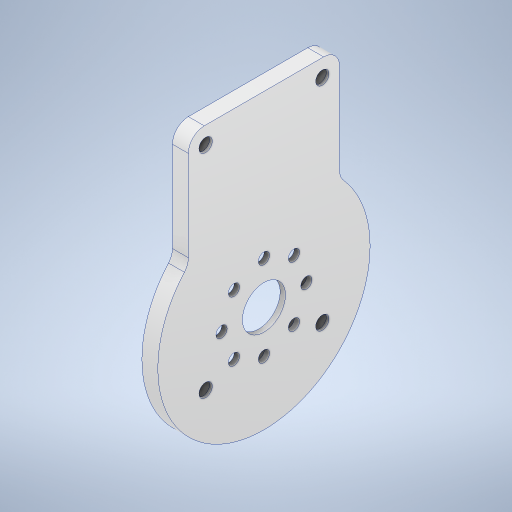
# Autodesk Inventor part: connectpart5
Saved by Autodesk Inventor 2024.3 (Build 283343010, 343A)
## iProperties
Created: 2025-06-29
Part Number: connectpart5
Material: アルミニウム 6061
Document SubType Name: Modeling
Designer: kshau
Density: 2.7 g/cm^3
Appearance: アルミニウム - フラット
Author: kshau
Autodesk Inventor part; units mm, degrees
ref_plane "YZ Plane" through (0, 0, 0) normal (1, 0, 0) x (0, 1, 0)
ref_plane "XZ Plane" through (0, 0, 0) normal (0, 1, 0) x (-1, 0, 0)
ref_plane "XY Plane" through (0, 0, 0) normal (0, 0, 1) x (1, 0, 0)
sketch "スケッチ1" plane through (0, 0, 0) normal (1, 0, 0) x (0, 1, 0)
  circle A0 centre (0, 0) radius 20
  circle A1 centre (0, 0) radius 9.75
  line L0 (0, 0) -> (35.25, 0)
  line L1 (35.25, 0) -> (35.25, -14.25)
  line L2 (35.25, -14.25) -> (0, -14.25)
  line L3 (0, -14.25) -> (0, 0)
  line L4 (35.25, 0) -> (35.25, 14.25)
  line L5 (35.25, 14.25) -> (0, 14.25)
  point P0 (14.0334, 14.25)
  point P1 (14.0334, -14.25)
  dimension "d0" = 40
  dimension "d1" = 19.5
  dimension "d2" = 14.25
  dimension "d3" = 35.25
  constraints: 12 end point, 2 centre point, 2 coincident, 2 parallel, 2 symmetric about line, 1 horizontal, 1 perpendicular
  measures "d0" diameter of A0
  measures "d1" diameter of A1
  measures "d2" distance of L0.end L1.end
  measures "d3" distance of L1.end L2.end
extrude "押し出し1" add sketch "スケッチ1" along normal blind 3
sketch "スケッチ2" plane through (0, 0, 0) normal (-1, 0, 0) x (0, 0, 1)
  arc A0 (-14.25, 14.0334) -> (14.25, 14.0334) centre (0, 0) ccw projected
  circle A1 centre (0, 0) radius 9.75
  dimension "d6" = 19.5
  constraints: 1 centre point, 1 coincident
  measures "d6" diameter of A1
extrude "押し出し2" cut sketch "スケッチ2" against normal blind 2
sketch "スケッチ3" plane through (2, 0, 0) normal (-1, 0, 0) x (0, 0, 1)
  circle A0 centre (0, 0) radius 8
  point P0 (0, 8)
  point P1 (-5.6569, 5.6569)
  point P2 (-8, 0)
  point P3 (-5.6569, -5.6569)
  point P4 (0, -8)
  point P5 (5.6569, -5.6569)
  point P6 (8, 0)
  point P7 (5.6569, 5.6569)
  dimension "d9" = 16
  dimension "d12" = 360
  constraints: 1 coincident, 1 vertical alignment, 11 other
hole "穴1" at (2, 8, 0) at (2, 5.6569, -5.6569) at (2, 0, -8) at (2, -5.6569, -5.6569) at (2, -8, 0) at (2, -5.6569, 5.6569) at (2, 0, 8) at (2, 5.6569, 5.6569) direction (1, 0, 0) diameter 2.1 end through all
sketch "スケッチ4" plane through (3, 0, 0) normal (1, 0, 0) x (0, 0, -1)
  line L0 (-14.25, 35.25) -> (-14.25, 14.0334) projected
  line L1 (-14.25, 35.25) -> (14.25, 35.25)
  line L2 (14.25, 35.25) -> (14.25, -11.25)
  line L3 (14.25, -11.25) -> (-14.25, -11.25)
  line L4 (-14.25, -11.25) -> (-14.25, 35.25)
  point P0 (0, 0)
  point P1 (-11, -8)
  point P2 (11, -8)
  point P3 (-11, 32)
  point P4 (11, 32)
  dimension "d21" = 46.5
  dimension "d22" = 3.25
  dimension "d23" = 3.25
  dimension "d24" = 3.25
  dimension "d25" = 3.25
  dimension "d26" = 3.25
  dimension "d27" = 3.25
  dimension "d28" = 3.25
  dimension "d29" = 3.25
  constraints: 8 end point, 2 parallel, 1 horizontal, 1 perpendicular, 1 point on line
  measures "d21" distance of L1.end L2.end
  measures "d22" distance from line of L2 point (11, -8)
  measures "d23" distance from line of L3 point (11, -8)
  measures "d24" distance from line of L4 point (-11, -8)
  measures "d25" distance from line of L3 point (-11, -8)
  measures "d26" distance from line of L0 point (-11, 32)
  measures "d27" distance from line of L1 point (-11, 32)
  measures "d28" distance from line of L1 point (11, 32)
  measures "d29" distance from line of L2 point (11, 32)
hole "穴2" at (3, -8, 11) at (3, -8, -11) at (3, 32, -11) at (3, 32, 11) direction (-1, 0, 0) diameter 2.5 end through all
sketch "スケッチ5" plane through (0, 0, 0) normal (-1, 0, 0) x (0, 0, 1)
  circle A0 centre (-11, -8) radius 1.25 projected
  circle A1 centre (-11, -8) radius 2.4
  circle A2 centre (11, -8) radius 1.25 projected
  circle A3 centre (11, -8) radius 2.4
  circle A4 centre (-11, 32) radius 1.25 projected
  circle A5 centre (-11, 32) radius 2.4
  circle A6 centre (11, 32) radius 1.25 projected
  circle A7 centre (11, 32) radius 2.4
  point P0 (0, 0)
  dimension "d37" = 4.8
  dimension "d38" = 4.8
  dimension "d39" = 4.8
  dimension "d40" = 4.8
  constraints: 4 centre point, 4 coincident
  measures "d37" diameter of A1
  measures "d38" diameter of A3
  measures "d39" diameter of A5
  measures "d40" diameter of A7
extrude "押し出し3" cut sketch "スケッチ5" against normal blind 2.5 contours A1 | A2 | A3 | A4 | A5 | A6 | A7
fillet "フィレット1" radius 3 4 edges at (1.5, 35.25, -14.25) (1.5, 35.25, 14.25) (1.5, 14.0334, -14.25) (1.5, 14.0334, 14.25)
sketch "スケッチ6" plane through (2, 0, 0) normal (-1, 0, 0) x (0, 0, 1)
  circle A0 centre (0, 0) radius 4.05
  dimension "d44" = 8.1
  constraints: 1 centre point, 1 coincident
  measures "d44" diameter of A0
extrude "押し出し4" cut sketch "スケッチ6" against normal blind 10
